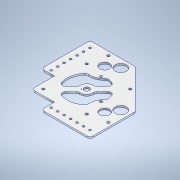
# Autodesk Inventor part: TopPlate
Saved by Autodesk Inventor 2020 (Build 240168000, 168)
## iProperties
Created: 2019-05-28
Part Number: TopPlate
Material: Aluminum 6061
Document SubType Name: Modeling
Designer: Connor
Density: 2.7 g/cm^3
Appearance: Aluminum - Flat
Author: Connor
Autodesk Inventor part; units mm, degrees
ref_plane "YZ Plane" through (0, 0, 0) normal (1, 0, 0) x (0, 1, 0)
ref_plane "XZ Plane" through (0, 0, 0) normal (0, 1, 0) x (-1, 0, 0)
ref_plane "XY Plane" through (0, 0, 0) normal (0, 0, 1) x (1, 0, 0)
sketch "Sketch1" plane through (0, 0, 0) normal (0, 1, 0) x (-1, 0, 0)
  line L0 (0, 0) -> (-165.1, 0)
  line L1 (-165.1, 0) -> (-165.1, -165.1)
  line L2 (-165.1, -165.1) -> (0, -165.1)
  line L3 (0, -165.1) -> (0, 0)
  circle A0 centre (-79.375, -79.375) radius 38.1
  line L4 (-25.4, -165.1) -> (-25.4, 0) construction
  line L5 (0, -25.4) -> (-165.1, -25.4) construction
  line L6 (0, 0) -> (-165.1, -165.1) construction
  circle A1 centre (-79.375, -79.375) radius 53.975 construction
  dimension "d0" = 76.2
  dimension "d3" = 25.4
  dimension "d4" = 25.4
  dimension "d5" = 107.95
  dimension "d25" = 165.1
  constraints: 14 end point, 7 point on line, 4 perpendicular, 2 centre point, 2 parallel, 1 coincident, 1 horizontal, 1 tangent
  measures "d0" diameter of A0
  measures "d3" distance between parallel lines of L0 L5
  measures "d4" distance between parallel lines of L3 L4
  measures "d5" diameter of A1
  measures "d25" distance between parallel lines of L0 L2
extrude "Extrusion1" add sketch "Sketch1" along normal blind 3.175
sketch "Sketch2" plane through (0, 3.175, 0) normal (0, 1, 0) x (1, 0, 0)
  circle A0 centre (79.375, 79.375) radius 38.1 construction
  circle A1 centre (79.375, 79.375) radius 60.325 construction
  line L0 (0, 165.1) -> (0, 0) construction
  arc A2 (184.15, 82.55) -> (82.55, 184.15) centre (82.55, 82.55) ccw construction
  line L1 (36.7188, 36.7188) -> (122.0312, 36.7188) construction
  line L2 (122.0312, 36.7188) -> (122.0312, 122.0312) construction
  line L3 (122.0312, 122.0312) -> (36.7188, 122.0312) construction
  line L4 (36.7188, 122.0312) -> (36.7188, 36.7188) construction
  dimension "d9" = 120.65
  constraints: 8 end point, 4 point on circle, 2 parallel, 2 perpendicular, 1 centre point, 1 coincident, 1 horizontal
  measures "d9" diameter of A1
hole "Hole1" at (36.7188, 3.175, -36.7188) at (122.0312, 3.175, -122.0312) at (122.0312, 3.175, -36.7188) at (36.7188, 3.175, -122.0312) direction (0, -1, 0) diameter 4.9784 end through all
sketch "Sketch3" plane through (0, 3.175, 0) normal (0, 1, 0) x (1, 0, 0)
  circle A0 centre (79.375, 79.375) radius 38.1 construction
  circle A1 centre (79.375, 79.375) radius 53.975 construction
  circle A2 centre (57.9215, 136.0171) radius 9.525
  line L0 (0, 0) -> (79.375, 79.375) construction
  circle A3 centre (136.0171, 57.9215) radius 9.525
  circle A4 centre (122.0312, 122.0312) radius 2.4892 construction
  circle A5 centre (57.9215, 136.0171) radius 22.86 construction
  line L1 (79.375, 79.375) -> (77.0039, 148.6044) construction
  circle A6 centre (77.0039, 148.6044) radius 11.1125
  circle A7 centre (148.6044, 77.0039) radius 11.1125
  circle A8 centre (57.9215, 136.0171) radius 25.4 construction
  circle A9 centre (122.0312, 122.0312) radius 4.7625 construction
  circle A10 centre (57.9215, 136.0171) radius 29.9974 construction
  circle A11 centre (36.7188, 122.0312) radius 2.4892 projected
  circle A12 centre (43.9356, 157.2198) radius 2.4892
  circle A13 centre (122.0312, 36.7188) radius 2.4892
  circle A14 centre (157.2198, 43.9356) radius 2.4892
  circle A15 centre (71.9074, 114.8144) radius 2.4892
  circle A16 centre (114.8144, 71.9074) radius 2.4892
  circle A17 centre (79.375, 79.375) radius 38.1 projected
  arc A18 (52.6128, 106.4932) -> (81.457, 117.4181) centre (57.9215, 136.0171) ccw
  arc A19 (117.4181, 81.457) -> (106.4932, 52.6128) centre (136.0171, 57.9215) ccw
  circle A20 centre (36.7188, 122.0312) radius 2.4892 projected
  line L2 (36.7188, 122.0312) -> (77.0039, 148.6044) construction
  point P0 (117.4181, 81.457)
  point P1 (106.4932, 52.6128)
  dimension "d33" = 45.72
  dimension "d17" = 107.95
  dimension "d19" = 19.05
  dimension "d34" = 69.27
  dimension "d35" = 22.225
  dimension "d37" = 50.8
  dimension "d38" = 59.9948
  dimension "d39" = 9.525
  dimension "d52" = 4.9784
  dimension "d53" = 90
  dimension "d56" = 90
  constraints: 15 centre point, 11 point on circle, 8 symmetric about line, 7 coincident, 6 end point, 1 equal radius, 1 point on line, 9 other
  measures "d17" diameter of A1
  measures "d19" diameter of A2
  measures "d34" distance of L0.end L1.end
  measures "d35" diameter of A6
  measures "d37" diameter of A8
  measures "d38" diameter of A10
  measures "d39" diameter of A9
  measures "d52" diameter of A12
extrude "Extrusion5" cut sketch "Sketch3" against normal through all contours A2 | A3 | A6 | A7 | A12 | A14 | A15 A17 | A17 A15 | A17 A16 | A16 A17
extrude "Extrusion6" add sketch "Sketch3" against normal up to surface (3.175 mm away) contours A15 A17 A18 | A17 A16 A19
sketch "Sketch5" plane through (0, 3.175, 0) normal (0, 1, 0) x (1, 0, 0)
  line L0 (0, 165.1) -> (0, 0) projected
  line L1 (0, 0) -> (25.4, 0)
  line L2 (25.4, 0) -> (25.4, 69.85)
  line L3 (25.4, 69.85) -> (0, 69.85)
  line L4 (0, 69.85) -> (0, 0)
  line L5 (25.4, 0) -> (69.85, 0)
  line L6 (69.85, 0) -> (69.85, 25.4)
  line L7 (69.85, 25.4) -> (25.4, 25.4)
  line L8 (25.4, 25.4) -> (25.4, 0)
  dimension "d63" = 25.4
  dimension "d64" = 69.85
  dimension "d65" = 44.45
  dimension "d66" = 25.4
  constraints: 16 end point, 4 parallel, 2 horizontal, 2 perpendicular
  measures "d63" distance of L3.end L2.end
  measures "d64" distance of L2.end L1.end
  measures "d65" distance of L7.end L6.end
  measures "d66" distance of L6.end L5.end
extrude "Extrusion7" cut sketch "Sketch5" against normal up to surface (3.175 mm away)
chamfer "Chamfer3" distance 76.2 angle 45 1 edges at (165.1, 1.5875, -165.1)
fillet "Fillet6" radius 6.35 7 edges at (165.1, 1.5875, 0) (165.1, 1.5875, -88.9) (88.9, 1.5875, -165.1) (0, 1.5875, -165.1) (25.4, 1.5875, -25.4) (0, 1.5875, -69.85) (69.85, 1.5875, 0)
sketch "Sketch6" plane through (0, 3.175, 0) normal (0, 1, 0) x (1, 0, 0)
  line L0 (0, 0) -> (12.7, 0) construction
  line L1 (12.7, 0) -> (12.7, 12.7) construction
  line L2 (12.7, 12.7) -> (0, 12.7) construction
  line L3 (0, 12.7) -> (0, 0) construction
  point P0 (25.4, 12.7)
  point P1 (38.1, 12.7)
  point P2 (50.8, 12.7)
  point P3 (63.5, 12.7)
  point P4 (76.2, 12.7)
  point P5 (88.9, 12.7)
  point P6 (101.6, 12.7)
  point P7 (114.3, 12.7)
  point P8 (127, 12.7)
  point P9 (139.7, 12.7)
  point P10 (152.4, 12.7)
  point P11 (12.7, 25.4)
  point P12 (12.7, 38.1)
  point P13 (12.7, 50.8)
  point P14 (12.7, 63.5)
  point P15 (12.7, 76.2)
  point P16 (12.7, 88.9)
  point P17 (12.7, 101.6)
  point P18 (12.7, 114.3)
  point P19 (12.7, 127)
  point P20 (12.7, 139.7)
  point P21 (12.7, 152.4)
  dimension "d77" = 12.7
  dimension "d78" = 12.7
  dimension "d81" = 12.7
  dimension "d88" = 12.7
  constraints: 8 end point, 2 horizontal, 2 parallel, 1 coincident, 1 perpendicular, 1 vertical, 22 other
  measures "d77" distance of L2.end L1.end
  measures "d78" distance of L1.end L0.end
  measures "d81" distance of point (12.7, 12.7) point (25.4, 12.7)
  measures "d88" distance of point (12.7, 12.7) point (12.7, 25.4)
hole "Hole2" at (12.7, 3.175, -12.7) at (25.4, 3.175, -12.7) at (38.1, 3.175, -12.7) at (50.8, 3.175, -12.7) at (63.5, 3.175, -12.7) at (76.2, 3.175, -12.7) at (88.9, 3.175, -12.7) at (101.6, 3.175, -12.7) at (114.3, 3.175, -12.7) at (127, 3.175, -12.7) at (139.7, 3.175, -12.7) at (152.4, 3.175, -12.7) at (12.7, 3.175, -25.4) at (12.7, 3.175, -38.1) at (12.7, 3.175, -50.8) at (12.7, 3.175, -63.5) at (12.7, 3.175, -76.2) at (12.7, 3.175, -88.9) at (12.7, 3.175, -101.6) at (12.7, 3.175, -114.3) at (12.7, 3.175, -127) at (12.7, 3.175, -139.7) at (12.7, 3.175, -152.4) direction (0, -1, 0) diameter 4.1402 end through all
sketch "Sketch7" plane through (0, 3.175, 0) normal (0, 1, 0) x (1, 0, 0)
  arc A0 (52.6128, 106.4932) -> (106.4932, 52.6128) centre (79.375, 79.375) ccw projected
  arc A1 (117.4181, 81.457) -> (81.457, 117.4181) centre (79.375, 79.375) ccw projected
  arc A2 (52.6128, 106.4932) -> (81.457, 117.4181) centre (57.9215, 136.0171) ccw projected
  arc A3 (117.4181, 81.457) -> (106.4932, 52.6128) centre (136.0171, 57.9215) ccw projected
  circle A4 centre (79.375, 79.375) radius 12.7
  line L0 (67.1077, 76.088) -> (76.088, 67.1077)
  line L1 (76.088, 67.1077) -> (57.3012, 48.3209)
  line L2 (57.3012, 48.3209) -> (48.3209, 57.3012)
  line L3 (48.3209, 57.3012) -> (67.1077, 76.088)
  circle A5 centre (36.7188, 36.7188) radius 2.4892 projected
  line L4 (79.375, 79.375) -> (36.7188, 36.7188) construction
  line L5 (101.4488, 110.4291) -> (110.4291, 101.4488)
  line L6 (110.4291, 101.4488) -> (91.6423, 82.662)
  line L7 (91.6423, 82.662) -> (82.662, 91.6423)
  line L8 (82.662, 91.6423) -> (101.4488, 110.4291)
  circle A6 centre (79.375, 79.375) radius 5.1562
  circle A7 centre (74.1665, 74.1665) radius 0.7874
  point P0 (0, 0)
  point P1 (48.3209, 57.3012)
  point P2 (48.3209, 57.3012)
  point P3 (110.4291, 101.4488)
  dimension "d100" = 25.4
  dimension "d102" = 12.7
  dimension "d106" = 10.3124
  dimension "d107" = 1.5748
  dimension "d108" = 7.366
  constraints: 18 end point, 6 point on circle, 5 parallel, 3 centre point, 2 coincident, 2 collinear, 2 perpendicular, 1 point on line
  measures "d100" diameter of A4
  measures "d102" distance between parallel lines of L1 L3
  measures "d106" diameter of A6
  measures "d107" diameter of A7
  measures "d108" distance of A7.centre A0.centre
extrude "Extrusion8" add sketch "Sketch7" against normal up to surface (3.175 mm away) contours L2 A0 | L3 A4 L1 L2 | L0 A4 | A4 L7 L0 | A1 L5 | L5 L6 A4 L8 | A4 L7
fillet "Fillet7" radius 6.35 12 edges at (76.088, 1.5875, -67.1077) (67.1077, 1.5875, -76.088) (48.3209, 1.5875, -57.3012) (57.3012, 1.5875, -48.3209) (110.4291, 1.5875, -101.4488) (101.4488, 1.5875, -110.4291) (82.662, 1.5875, -91.6423) (91.6423, 1.5875, -82.662) (52.6128, 1.5875, -106.4932) (81.457, 1.5875, -117.4181) (106.4932, 1.5875, -52.6128) (117.4181, 1.5875, -81.457)
body "Solid1"
